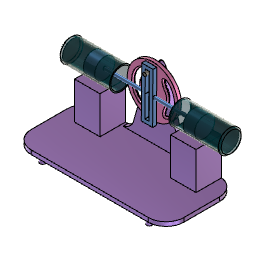
Yoke Mechanism (Autodesk Fusion 360 design; units mm, degrees)
Autodesk Fusion 360 part; units mm, degrees
note: some values were not read from the file. Set by a fixed rule: which face or edge a step refers to.
sketch "stand bottom" plane through (0, 0, 0) normal (0, 0, 1) x (1, 0, 0) in component "Stand"
  line L0 (150, 70) -> (-150, 70)
  line L1 (-150, 70) -> (-150, -70)
  line L2 (-150, -70) -> (150, -70)
  line L3 (150, -70) -> (150, 70)
  circle A0 centre (-105, 58) radius 5
  circle A1 centre (-105, -58) radius 5
  circle A2 centre (105, 58) radius 5
  circle A3 centre (105.0261, -58) radius 5
  dimension "d1" = 10
  dimension "d4" = 10
  dimension "d5" = 10
  dimension "d6" = 10
  constraint horizontal L0
  constraint vertical L1
  constraint horizontal L2
  constraint vertical L3
  measures "d1" diameter of A0
  measures "d4" diameter of A1
  measures "d5" diameter of A2
  measures "d6" diameter of A3
extrude "Extrude1" add sketch "stand bottom" along normal blind 8 contours L0 L1 L2 L3 | A0 | A1 | A2 | A3 makes body 1 in component "Stand"
extrude "Extrude2" add sketch "stand bottom" against normal blind 14 contours A0 | A1 | A2 | A3 bodies 1 in component "Stand"
fillet "Fillet1" radius 35 4 edges at (-150, 70, 4) (150, 70, 4) (150, -70, 4) (-150, -70, 4) on bodies 1 in component "Stand"
sketch "stand top" plane through (0, 70, 0) normal (0, 1, 0) x (-1, 0, 0) in component "Stand"
  line L0 (-115, 8) -> (-115, 0)
  line L1 (-115, 0) -> (115, 0)
  line L2 (115, 0) -> (115, 8)
  line L3 (115, 8) -> (-115, 8)
  line L4 (-50, 8) -> (50, 8)
  line L5 (-1.9252, 149.8221) -> (-2.2092, 149.8221)
  spline S0 degree 5 poles (-64.9527, 8) (-64.3612, 8.1995) (-63.1954, 8.61) (-61.498, 9.2603) (-59.339, 10.1978) (-56.826, 11.4952) (-54.5169, 12.9303) (-52.4304, 14.5157) (-50.5804, 16.2608) (-48.9632, 18.1632) (-47.5635, 20.2124) (-46.6045, 21.9603) (-45.9702, 23.3287) (-45.5844, 24.2659) (-45.4008, 24.7409) knots 0 0 0 0 0 0 0.1 0.2 0.3 0.4 0.5 0.6 0.7 0.8 0.9 1 1 1 1 1 1
  spline S1 degree 5 poles (65.0799, 8) (64.5003, 8.2031) (63.3571, 8.6206) (61.69, 9.2805) (59.5642, 10.2292) (57.0799, 11.5375) (54.785, 12.98) (52.6968, 14.5689) (50.8278, 16.3131) (49.1739, 18.2095) (47.7205, 20.248) (46.7061, 21.9839) (46.0235, 23.3412) (45.6026, 24.2703) (45.4008, 24.7409) knots 0 0 0 0 0 0 0.1 0.2 0.3 0.4 0.5 0.6 0.7 0.8 0.9 1 1 1 1 1 1
  line L6 (-64.9527, 8) -> (65.0799, 8)
  spline S2 degree 5 poles (-45.4008, 24.7409) (-42.8881, 33.5033) (-38.082, 50.4523) (-31.5308, 74.1483) (-24.0174, 102.0268) (-16.1362, 129.1634) (-9.099, 146.6861) (-2.2181, 152.8633) (5.106, 146.8269) (13.2741, 129.4242) (22.5509, 102.341) (30.9962, 74.4151) (37.9521, 50.6146) (42.871, 33.5629) (45.4008, 24.7408) knots 0 0 0 0 0 0 0.1 0.2 0.3 0.4 0.5 0.6 0.7 0.8 0.9 1 1 1 1 1 1
  line L7 (-51.345, 4.0119) -> (-39.4565, 45.4698)
  line L8 (39.4565, 45.4698) -> (51.345, 4.0119)
  point P0 (-51.9875, 14.9922)
  point P1 (52.3054, 14.9922)
  dimension "d14" = 100
  constraint horizontal L4
  constraint horizontal L5
  constraint coincident L3 S0.start
  constraint coincident L3 S1.start
  constraint coincident S1.end S2
  constraint coincident S1 S2.end
  constraint midpoint S0.end L7
  constraint midpoint S2.end L8
  constraint coincident S2 L5.start
  measures "d14" distance of L4.start L4.end
extrude "Extrude3" add sketch "stand top" against normal blind 10 contours L3 S0 L6 L7 | L3 L4 L5 L6 S2 L7 L8 | L3 S1 L6 L8 bodies 1 in component "Stand"
sketch "crank holes" plane through (0, 60, 0) normal (0, -1, 0) x (1, 0, 0) in component "Crank"
  line L0 (-65.0799, 8) -> (64.9527, 8)
  spline S0 degree 5 poles (64.9527, 8) (64.3612, 8.1995) (63.1954, 8.61) (61.498, 9.2603) (59.339, 10.1978) (56.826, 11.4952) (54.5169, 12.9303) (52.4304, 14.5157) (50.5804, 16.2608) (48.9632, 18.1632) (47.5635, 20.2124) (46.6045, 21.9603) (45.9702, 23.3287) (45.5844, 24.2659) (45.4008, 24.7409) knots 0 0 0 0 0 0 0.1 0.2 0.3 0.4 0.5 0.6 0.7 0.8 0.9 1 1 1 1 1 1
  spline S1 degree 5 poles (45.4008, 24.7409) (42.8881, 33.5033) (38.082, 50.4523) (31.5308, 74.1483) (24.0174, 102.0268) (16.1583, 129.0872) (10.546, 143.0831) (6.4127, 148.5135) (3.6169, 149.7753) (2.2092, 149.8221) knots 0 0 0 0 0 0 0.1 0.2 0.3 0.4 0.498596 0.498596 0.498596 0.498596 0.498596 0.498596
  line L1 (2.2092, 149.8221) -> (1.9252, 149.8221)
  spline S2 degree 5 poles (-45.4008, 24.7409) (-45.6026, 24.2703) (-46.0235, 23.3412) (-46.7061, 21.9839) (-47.7205, 20.248) (-49.1739, 18.2095) (-50.8278, 16.3131) (-52.6968, 14.5689) (-54.785, 12.98) (-57.0799, 11.5375) (-59.5642, 10.2292) (-61.69, 9.2805) (-63.3571, 8.6206) (-64.5003, 8.2031) (-65.0799, 8) knots -1 -1 -1 -1 -1 -1 -0.9 -0.8 -0.7 -0.6 -0.5 -0.4 -0.3 -0.2 -0.1 0 0 0 0 0 0
  spline S3 degree 5 poles (-30, 90) (-30.1222, 90.4299) (-30.1922, 91.398) (-29.7437, 93.1541) (-27.9759, 95.973) (-23.8911, 99.8217) (-18.1874, 103.4577) (-11.2539, 106.3526) (-3.5648, 108.0684) (4.367, 108.3276) (12.0396, 107.1126) (18.9937, 104.6588) (24.8283, 101.3641) (29.2216, 97.7238) (31.9508, 94.2565) (32.9127, 91.4333) (32.146, 89.6068) (29.8541, 88.9368) (26.3462, 89.3976) (21.972, 90.7776) (17.0724, 92.7047) (11.9619, 94.7305) (6.9054, 96.4005) (2.0938, 97.3326) (-2.3738, 97.2842) (-6.5262, 96.2467) (-10.4934, 94.4463) (-14.4197, 92.253) (-18.388, 90.114) (-22.3503, 88.4802) (-26.0299, 87.7313) (-28.3367, 88.0383) (-29.4588, 88.8188) (-29.8778, 89.5701) (-30, 90) knots 0 0 0 0 0 0 0.033333 0.066667 0.1 0.133333 0.166667 0.2 0.233333 0.266667 0.3 0.333333 0.366667 0.4 0.433333 0.466667 0.5 0.533333 0.566667 0.6 0.633333 0.666667 0.7 0.733333 0.766667 0.8 0.833333 0.866667 0.9 0.933333 0.966667 1 1 1 1 1 1
  spline S4 degree 5 poles (31.4369, 46.3788) (31.5413, 45.9359) (31.5774, 44.9363) (31.0882, 43.1175) (29.2976, 40.1923) (25.2372, 36.2169) (19.5947, 32.514) (12.737, 29.663) (5.1206, 28.1374) (-2.7442, 28.2233) (-10.33, 29.9039) (-17.1277, 32.8669) (-22.6835, 36.6203) (-26.6352, 40.5748) (-28.7502, 44.14) (-28.9632, 46.8127) (-27.4177, 48.2723) (-24.5009, 48.4663) (-20.7069, 47.5475) (-16.5203, 45.8198) (-12.2699, 43.683) (-8.1234, 41.5748) (-4.1345, 39.9118) (-0.2722, 39.028) (3.5427, 39.1206) (7.4052, 40.1744) (11.3918, 41.9656) (15.5288, 44.1399) (19.7568, 46.269) (23.902, 47.9142) (27.6282, 48.6884) (29.8854, 48.3891) (30.9509, 47.5938) (31.3325, 46.8217) (31.4369, 46.3788) knots 0 0 0 0 0 0 0.033333 0.066667 0.1 0.133333 0.166667 0.2 0.233333 0.266667 0.3 0.333333 0.366667 0.4 0.433333 0.466667 0.5 0.533333 0.566667 0.6 0.633333 0.666667 0.7 0.733333 0.766667 0.8 0.833333 0.866667 0.9 0.933333 0.966667 1 1 1 1 1 1
  spline S5 degree 5 poles (1.9252, 149.8221) (0.531, 149.7759) (-2.3348, 148.5351) (-6.8236, 143.1672) (-13.3217, 129.285) (-22.5509, 102.341) (-30.9962, 74.4151) (-37.9521, 50.6146) (-42.871, 33.5629) (-45.4008, 24.7409) knots 0.50257 0.50257 0.50257 0.50257 0.50257 0.50257 0.6 0.7 0.8 0.9 1 1 1 1 1 1
  point P0 (0, 108)
  point P1 (32.484, 91.6271)
  point P2 (27.3786, 89.3794)
  point P3 (-0.1137, 97.1853)
  point P4 (-21.072, 89.1079)
  point P5 (-28.5631, 46.3788)
  point P6 (-19.4459, 46.9397)
  point P7 (1.4369, 28.3788)
  point P8 (22.5089, 47.2709)
  point P9 (1.5506, 39.1935)
  constraint coincident S1 P2
sketch "crank" plane through (0, 60, 0) normal (0, -1, 0) x (1, 0, 0) in component "Crank"
  circle A0 centre (0.0497, 67.3306) radius 50
  dimension "d19" = 100
  measures "d19" diameter of A0
extrude "Extrude1'" add sketch "crank" along normal blind 6.5 separate body makes body 2 in component "Crank"
extrude "Extrude2'" cut sketch "crank holes" along normal blind 20 contours S1 S3 S5 | S3 S5 | S1 S3 | S4 bodies 2 in component "Crank"
fillet "Fillet1'" radius 2.5 1 faces at (19.1682, 57.8333, 91.8987) on bodies 2 in component "Crank"
fillet "Fillet2" radius 2.5 1 faces at (12.9137, 55.6667, 42.7911) on bodies 2 in component "Crank"
sketch "crank pin" plane through (0, 53.5, 0) normal (0, -1, 0) x (1, 0, 0) in component "Crank"
  spline S0 degree 3 poles (-32.4047, 89.3162) (-32.2002, 88.597) (-31.8287, 87.9253) (-30.5196, 86.4929) (-29.397, 85.9429) (-27.7418, 85.5869) (-27.2429, 85.5296) (-25.5741, 85.4613) (-24.4031, 85.6084) (-22.117, 86.1062) (-20.9991, 86.4599) (-18.0884, 87.5643) (-16.3403, 88.4246) (-12.8647, 90.2551) (-11.1373, 91.2339) (-8.0614, 92.7587) (-6.7334, 93.3488) (-3.982, 94.2439) (-2.5577, 94.5401) (0.5399, 94.7607) (2.2064, 94.6297) (6.2945, 93.9154) (8.6805, 93.1627) (12.6221, 91.7573) (14.2021, 91.1432) (17.2778, 89.946) (18.7736, 89.3612) (21.6215, 88.3307) (22.9694, 87.8752) (25.3002, 87.237) (26.2721, 87.0129) (28.5577, 86.6781) (29.8981, 86.6164) (31.6823, 87.0406) (32.1742, 87.2205) (33.458, 87.9311) (34.1502, 88.6448) (34.8897, 90.2302) (35.0207, 91.0446) (34.9052, 93.1494) (34.4037, 94.3994) (32.8586, 97.0913) (31.6734, 98.4685) (29.0957, 100.9728) (27.6888, 102.0975) (22.8051, 105.4634) (19.0241, 107.252) (11.0474, 109.7644) (6.8251, 110.452) (-0.3594, 110.5842) (-3.3171, 110.3429) (-9.1325, 109.2942) (-11.9883, 108.4886) (-16.7168, 106.6518) (-18.6397, 105.7493) (-21.906, 103.9112) (-23.2799, 103.0321) (-25.4581, 101.4258) (-26.2992, 100.7465) (-27.9744, 99.2379) (-28.8028, 98.401) (-30.1414, 96.809) (-30.6813, 96.079) (-31.4524, 94.8032) (-31.7251, 94.2831) (-32.2133, 93.1239) (-32.4148, 92.4775) (-32.6035, 91.3035) (-32.6287, 90.7829) (-32.5513, 89.9463) (-32.4931, 89.627) (-32.4047, 89.3162) knots -36.87303517 -36.87303517 -36.87303517 -36.87303517 -36.59704222 -36.59704222 -36.15680654 -36.15680654 -35.97209665 -35.97209665 -35.54026559 -35.54026559 -35.10843452 -35.10843452 -34.39112682 -34.39112682 -33.65770849 -33.65770849 -33.12392068 -33.12392068 -32.59012672 -32.59012672 -31.97764095 -31.97764095 -31.05827941 -31.05827941 -30.43187642 -30.43187642 -29.83920987 -29.83920987 -29.31415769 -29.31415769 -28.94687666 -28.94687666 -28.4615352 -28.4615352 -28.26997051 -28.26997051 -27.91990285 -27.91990285 -27.62431801 -27.62431801 -27.14178902 -27.14178902 -26.47846917 -26.47846917 -25.81514933 -25.81514933 -24.2891365 -24.2891365 -22.72668726 -22.72668726 -21.63678991 -21.63678991 -20.54546925 -20.54546925 -19.76392124 -19.76392124 -19.16273047 -19.16273047 -18.76364224 -18.76364224 -18.33039407 -18.33039407 -17.99617584 -17.99617584 -17.77997858 -17.77997858 -17.53188563 -17.53188563 -17.34104489 -17.34104489 -17.22176943 -17.22176943 -17.22176943 -17.22176943
  circle A0 centre (0.0497, 67.3306) radius 50
  spline S1 degree 3 poles (33.8702, 46.9525) (33.7673, 47.3887) (33.6068, 47.8118) (33.0061, 48.8977) (32.4431, 49.4885) (31.0994, 50.3592) (30.3223, 50.6347) (28.791, 50.9139) (28.0381, 50.9408) (26.3548, 50.8495) (25.4262, 50.694) (22.2649, 49.9512) (20.1088, 49.0782) (16.5392, 47.4347) (15.095, 46.7026) (12.1973, 45.2273) (10.7441, 44.4811) (8.5258, 43.4711) (7.7841, 43.1548) (5.7652, 42.3957) (4.4602, 42.0117) (2.2222, 41.6956) (1.31, 41.6594) (-0.503, 41.7823) (-1.402, 41.9396) (-4.2235, 42.6592) (-6.0723, 43.4581) (-9.5174, 45.0826) (-11.1252, 45.9081) (-13.7245, 47.1836) (-14.7078, 47.6541) (-17.001, 48.6799) (-18.3199, 49.2195) (-20.5724, 49.97) (-21.4888, 50.2307) (-23.3369, 50.6129) (-24.2699, 50.7381) (-26.2035, 50.747) (-27.2125, 50.6101) (-28.6325, 50.0197) (-29.1022, 49.7395) (-30.014, 48.9559) (-30.4226, 48.4155) (-30.9212, 47.3276) (-31.0582, 46.8033) (-31.1858, 45.5883) (-31.1253, 44.8947) (-30.7455, 43.198) (-30.3147, 42.225) (-29.4705, 40.7504) (-29.1117, 40.21) (-27.8354, 38.4776) (-26.8112, 37.369) (-23.6636, 34.4157) (-21.3575, 32.7687) (-15.5428, 29.4373) (-11.8892, 27.9817) (-5.984, 26.5351) (-3.8202, 26.1833) (1.6474, 25.744) (4.9692, 25.8858) (10.4357, 26.7953) (12.6173, 27.3464) (16.9342, 28.8183) (19.0646, 29.7497) (22.5636, 31.6522) (23.9796, 32.5395) (26.5538, 34.4097) (27.7243, 35.3757) (29.5534, 37.1373) (30.2557, 37.8879) (31.5452, 39.4688) (32.1351, 40.2986) (33.0522, 41.9092) (33.4076, 42.6746) (33.8719, 44.1661) (34.0067, 44.8845) (34.0192, 46.0595) (33.9739, 46.5126) (33.8702, 46.9525) knots -50.17481759 -50.17481759 -50.17481759 -50.17481759 -49.94582152 -49.94582152 -49.54091284 -49.54091284 -49.12785412 -49.12785412 -48.74565958 -48.74565958 -48.26666293 -48.26666293 -47.08607969 -47.08607969 -46.25822908 -46.25822908 -45.4243524 -45.4243524 -45.01222338 -45.01222338 -44.32140201 -44.32140201 -43.85749851 -43.85749851 -43.39359501 -43.39359501 -42.36995809 -42.36995809 -41.44707773 -41.44707773 -40.88986856 -40.88986856 -40.16336921 -40.16336921 -39.67695209 -39.67695209 -39.19871179 -39.19871179 -38.68910161 -38.68910161 -38.41314855 -38.41314855 -38.07490321 -38.07490321 -37.80173618 -37.80173618 -37.45077222 -37.45077222 -36.91346781 -36.91346781 -36.58272177 -36.58272177 -35.81423378 -35.81423378 -34.37765011 -34.37765011 -32.38849479 -32.38849479 -31.27192126 -31.27192126 -29.58592663 -29.58592663 -28.44053696 -28.44053696 -27.25640945 -27.25640945 -26.40408789 -26.40408789 -25.6313644 -25.6313644 -25.10672795 -25.10672795 -24.58857947 -24.58857947 -24.15996572 -24.15996572 -23.79053685 -23.79053685 -23.5596438 -23.5596438 -23.5596438 -23.5596438
  circle A1 centre (-36.403, 67.3306) radius 4
  arc A2 (31.9944, 49.771) -> (31.9946, 49.7712) centre (0.0497, 67.3306) ccw
  arc A3 (30.8161, 86.8814) -> (30.816, 86.8814) centre (0.0497, 67.3306) ccw
  dimension "d28" = 8
  constraint coincident S1 A2.end
  constraint coincident S0 A3.start
  constraint coincident S1 A2.start
  constraint coincident S0 A3.end
  measures "d28" diameter of A1
extrude "Extrude3'" add sketch "crank pin" along normal blind 16 and the other way blind 5 separate body contours A1 A2 A3 | A1 A2 A3 makes body 3 in component "Crank"
sketch "stand pin" plane through (0, 60, 0) normal (0, -1, 0) x (1, 0, 0) in component "Stand"
  line L0 (-65.0799, 8) -> (64.9527, 8)
  spline S0 degree 5 poles (64.9527, 8) (64.3612, 8.1995) (63.1954, 8.61) (61.498, 9.2603) (59.339, 10.1978) (56.826, 11.4952) (54.5169, 12.9303) (52.4304, 14.5157) (50.5804, 16.2608) (48.9632, 18.1632) (47.5635, 20.2124) (46.6045, 21.9603) (45.9702, 23.3287) (45.5844, 24.2659) (45.4008, 24.7409) knots 0 0 0 0 0 0 0.1 0.2 0.3 0.4 0.5 0.6 0.7 0.8 0.9 1 1 1 1 1 1
  spline S1 degree 5 poles (45.4008, 24.7409) (42.8881, 33.5033) (38.082, 50.4523) (31.5308, 74.1483) (24.0174, 102.0268) (16.1583, 129.0872) (10.546, 143.0831) (6.4127, 148.5135) (3.6169, 149.7753) (2.2092, 149.8221) knots 0 0 0 0 0 0 0.1 0.2 0.3 0.4 0.498596 0.498596 0.498596 0.498596 0.498596 0.498596
  line L1 (2.2092, 149.8221) -> (1.9252, 149.8221)
  spline S2 degree 5 poles (-45.4008, 24.7409) (-45.6026, 24.2703) (-46.0235, 23.3412) (-46.7061, 21.9839) (-47.7205, 20.248) (-49.1739, 18.2095) (-50.8278, 16.3131) (-52.6968, 14.5689) (-54.785, 12.98) (-57.0799, 11.5375) (-59.5642, 10.2292) (-61.69, 9.2805) (-63.3571, 8.6206) (-64.5003, 8.2031) (-65.0799, 8) knots -1 -1 -1 -1 -1 -1 -0.9 -0.8 -0.7 -0.6 -0.5 -0.4 -0.3 -0.2 -0.1 0 0 0 0 0 0
  circle A0 centre (1.5, 104) radius 3
  spline S3 degree 5 poles (1.9252, 149.8221) (0.531, 149.7759) (-2.3348, 148.5351) (-6.8236, 143.1672) (-13.3217, 129.285) (-22.5509, 102.341) (-30.9962, 74.4151) (-37.9521, 50.6146) (-42.871, 33.5629) (-45.4008, 24.7409) knots 0.50257 0.50257 0.50257 0.50257 0.50257 0.50257 0.6 0.7 0.8 0.9 1 1 1 1 1 1
  dimension "d34" = 6
  measures "d34" diameter of A0
extrude "Extrude4" cut sketch "stand pin" against normal blind 0.7 bodies 1 in component "Stand"
extrude "Extrude5" add 1 faces at (3.554, 60, 103.4545) along direction (0, -1, 0) blind 10 and the other way blind 10 on bodies 1 bodies 1 in component "Stand"
sketch "crank middle hole" plane through (0, 53.5, 0) normal (0, -1, 0) x (1, 0, 0) in component "Crank"
  spline S0 degree 3 poles (-32.4047, 89.3162) (-32.2002, 88.597) (-31.8287, 87.9253) (-30.5196, 86.4929) (-29.397, 85.9429) (-27.7418, 85.5869) (-27.2429, 85.5296) (-25.5741, 85.4613) (-24.4031, 85.6084) (-22.117, 86.1062) (-20.9991, 86.4599) (-18.0884, 87.5643) (-16.3403, 88.4246) (-12.8647, 90.2551) (-11.1373, 91.2339) (-8.0614, 92.7587) (-6.7334, 93.3488) (-3.982, 94.2439) (-2.5577, 94.5401) (0.5399, 94.7607) (2.2064, 94.6297) (6.2945, 93.9154) (8.6805, 93.1627) (12.6221, 91.7573) (14.2021, 91.1432) (17.2778, 89.946) (18.7736, 89.3612) (21.6215, 88.3307) (22.9694, 87.8752) (25.3002, 87.237) (26.2721, 87.0129) (28.5577, 86.6781) (29.8981, 86.6164) (31.6823, 87.0406) (32.1742, 87.2205) (33.458, 87.9311) (34.1502, 88.6448) (34.8897, 90.2302) (35.0207, 91.0446) (34.9052, 93.1494) (34.4037, 94.3994) (32.8586, 97.0913) (31.6734, 98.4685) (29.0957, 100.9728) (27.6888, 102.0975) (22.8051, 105.4634) (19.0241, 107.252) (11.0474, 109.7644) (6.8251, 110.452) (-0.3594, 110.5842) (-3.3171, 110.3429) (-9.1325, 109.2942) (-11.9883, 108.4886) (-16.7168, 106.6518) (-18.6397, 105.7493) (-21.906, 103.9112) (-23.2799, 103.0321) (-25.4581, 101.4258) (-26.2992, 100.7465) (-27.9744, 99.2379) (-28.8028, 98.401) (-30.1414, 96.809) (-30.6813, 96.079) (-31.4524, 94.8032) (-31.7251, 94.2831) (-32.2133, 93.1239) (-32.4148, 92.4775) (-32.6035, 91.3035) (-32.6287, 90.7829) (-32.5513, 89.9463) (-32.4931, 89.627) (-32.4047, 89.3162) knots -36.87303517 -36.87303517 -36.87303517 -36.87303517 -36.59704222 -36.59704222 -36.15680654 -36.15680654 -35.97209665 -35.97209665 -35.54026559 -35.54026559 -35.10843452 -35.10843452 -34.39112682 -34.39112682 -33.65770849 -33.65770849 -33.12392068 -33.12392068 -32.59012672 -32.59012672 -31.97764095 -31.97764095 -31.05827941 -31.05827941 -30.43187642 -30.43187642 -29.83920987 -29.83920987 -29.31415769 -29.31415769 -28.94687666 -28.94687666 -28.4615352 -28.4615352 -28.26997051 -28.26997051 -27.91990285 -27.91990285 -27.62431801 -27.62431801 -27.14178902 -27.14178902 -26.47846917 -26.47846917 -25.81514933 -25.81514933 -24.2891365 -24.2891365 -22.72668726 -22.72668726 -21.63678991 -21.63678991 -20.54546925 -20.54546925 -19.76392124 -19.76392124 -19.16273047 -19.16273047 -18.76364224 -18.76364224 -18.33039407 -18.33039407 -17.99617584 -17.99617584 -17.77997858 -17.77997858 -17.53188563 -17.53188563 -17.34104489 -17.34104489 -17.22176943 -17.22176943 -17.22176943 -17.22176943
  circle A0 centre (0.0497, 67.3306) radius 50
  spline S1 degree 3 poles (33.8702, 46.9525) (33.7673, 47.3887) (33.6068, 47.8118) (33.0061, 48.8977) (32.4431, 49.4885) (31.0994, 50.3592) (30.3223, 50.6347) (28.791, 50.9139) (28.0381, 50.9408) (26.3548, 50.8495) (25.4262, 50.694) (22.2649, 49.9512) (20.1088, 49.0782) (16.5392, 47.4347) (15.095, 46.7026) (12.1973, 45.2273) (10.7441, 44.4811) (8.5258, 43.4711) (7.7841, 43.1548) (5.7652, 42.3957) (4.4602, 42.0117) (2.2222, 41.6956) (1.31, 41.6594) (-0.503, 41.7823) (-1.402, 41.9396) (-4.2235, 42.6592) (-6.0723, 43.4581) (-9.5174, 45.0826) (-11.1252, 45.9081) (-13.7245, 47.1836) (-14.7078, 47.6541) (-17.001, 48.6799) (-18.3199, 49.2195) (-20.5724, 49.97) (-21.4888, 50.2307) (-23.3369, 50.6129) (-24.2699, 50.7381) (-26.2035, 50.747) (-27.2125, 50.6101) (-28.6325, 50.0197) (-29.1022, 49.7395) (-30.014, 48.9559) (-30.4226, 48.4155) (-30.9212, 47.3276) (-31.0582, 46.8033) (-31.1858, 45.5883) (-31.1253, 44.8947) (-30.7455, 43.198) (-30.3147, 42.225) (-29.4705, 40.7504) (-29.1117, 40.21) (-27.8354, 38.4776) (-26.8112, 37.369) (-23.6636, 34.4157) (-21.3575, 32.7687) (-15.5428, 29.4373) (-11.8892, 27.9817) (-5.984, 26.5351) (-3.8202, 26.1833) (1.6474, 25.744) (4.9692, 25.8858) (10.4357, 26.7953) (12.6173, 27.3464) (16.9342, 28.8183) (19.0646, 29.7497) (22.5636, 31.6522) (23.9796, 32.5395) (26.5538, 34.4097) (27.7243, 35.3757) (29.5534, 37.1373) (30.2557, 37.8879) (31.5452, 39.4688) (32.1351, 40.2986) (33.0522, 41.9092) (33.4076, 42.6746) (33.8719, 44.1661) (34.0067, 44.8845) (34.0192, 46.0595) (33.9739, 46.5126) (33.8702, 46.9525) knots -50.17481759 -50.17481759 -50.17481759 -50.17481759 -49.94582152 -49.94582152 -49.54091284 -49.54091284 -49.12785412 -49.12785412 -48.74565958 -48.74565958 -48.26666293 -48.26666293 -47.08607969 -47.08607969 -46.25822908 -46.25822908 -45.4243524 -45.4243524 -45.01222338 -45.01222338 -44.32140201 -44.32140201 -43.85749851 -43.85749851 -43.39359501 -43.39359501 -42.36995809 -42.36995809 -41.44707773 -41.44707773 -40.88986856 -40.88986856 -40.16336921 -40.16336921 -39.67695209 -39.67695209 -39.19871179 -39.19871179 -38.68910161 -38.68910161 -38.41314855 -38.41314855 -38.07490321 -38.07490321 -37.80173618 -37.80173618 -37.45077222 -37.45077222 -36.91346781 -36.91346781 -36.58272177 -36.58272177 -35.81423378 -35.81423378 -34.37765011 -34.37765011 -32.38849479 -32.38849479 -31.27192126 -31.27192126 -29.58592663 -29.58592663 -28.44053696 -28.44053696 -27.25640945 -27.25640945 -26.40408789 -26.40408789 -25.6313644 -25.6313644 -25.10672795 -25.10672795 -24.58857947 -24.58857947 -24.15996572 -24.15996572 -23.79053685 -23.79053685 -23.5596438 -23.5596438 -23.5596438 -23.5596438
  circle A1 centre (0.0497, 67.3306) radius 3
  dimension "d41" = 6
  constraint concentric A0 A1
  measures "d41" diameter of A1
extrude "Extrude4'" cut 1 faces at (3.554, 50, 103.4545) along direction (0, 1, 0) blind 100 on bodies 1 bodies 3 2 in component "Crank"
move_face "OffsetFaces1" offset -0.3 1 faces at (4.3191, 57.1333, 102.9739) on bodies 1 in component "Stand"
sketch "left cylinder" plane through (-150, 0, 0) normal (-1, 0, 0) x (0, -1, 0) in component "Cylinders"
  line L0 (35, 0) -> (35, 8)
  line L1 (35, 8) -> (-35, 8)
  line L2 (-35, 8) -> (-35, 0)
  line L3 (-35, 0) -> (35, 0)
  circle A0 centre (10, 70) radius 22.5
  dimension "d45" = 45
  measures "d45" diameter of A0
extrude "Extrude1''" add sketch "left cylinder" against normal blind 100 separate body contours A0 makes body 4 in component "Cylinders"
sketch "left cylinder hole" plane through (-50, 0, 0) normal (1, 0, 0) x (0, 1, 0) in component "Cylinders"
  circle A0 centre (-10, 70) radius 22.5
  circle A1 centre (-10, 70) radius 20
  dimension "d48" = 40
  constraint concentric A0 A1
  measures "d48" diameter of A1
extrude "Extrude2''" cut sketch "left cylinder hole" against normal blind 95 contours A1 bodies 4 in component "Cylinders"
sketch "right cylinder" plane through (130.7682, 0, 0) normal (1, 0, 0) x (0, 1, 0) in component "Cylinders"
  line L0 (-66.6038, 25.1959) -> (-66.6038, 17.1959)
  line L1 (-66.6038, 17.1959) -> (3.3962, 17.1959)
  line L2 (3.3962, 17.1959) -> (3.3962, 25.1959)
  line L3 (3.3962, 25.1959) -> (-66.6038, 25.1959)
  circle A0 centre (-10, 70) radius 22.5
  dimension "d51" = 45
  measures "d51" diameter of A0
extrude "Extrude3''" add sketch "right cylinder" against normal blind 100 separate body contours A0 makes body 5 in component "Cylinders"
sketch "right cylinder hole" plane through (30.7682, 0, 0) normal (-1, 0, 0) x (0, -1, 0) in component "Cylinders"
  circle A0 centre (10, 70) radius 22.5
  circle A1 centre (10, 70) radius 20
  dimension "d54" = 40
  constraint concentric A0 A1
  measures "d54" diameter of A1
extrude "Extrude4''" cut sketch "right cylinder hole" against normal blind 95 contours A1 bodies 5 in component "Cylinders"
sketch "piston middle" plane through (0, 53.5, 0) normal (0, -1, 0) x (1, 0, 0) in component "Piston"
  spline S0 degree 3 poles (-32.4047, 89.3162) (-32.2002, 88.597) (-31.8287, 87.9253) (-30.5196, 86.4929) (-29.397, 85.9429) (-27.7418, 85.5869) (-27.2429, 85.5296) (-25.5741, 85.4613) (-24.4031, 85.6084) (-22.117, 86.1062) (-20.9991, 86.4599) (-18.0884, 87.5643) (-16.3403, 88.4246) (-12.8647, 90.2551) (-11.1373, 91.2339) (-8.0614, 92.7587) (-6.7334, 93.3488) (-3.982, 94.2439) (-2.5577, 94.5401) (0.5399, 94.7607) (2.2064, 94.6297) (6.2945, 93.9154) (8.6805, 93.1627) (12.6221, 91.7573) (14.2021, 91.1432) (17.2778, 89.946) (18.7736, 89.3612) (21.6215, 88.3307) (22.9694, 87.8752) (25.3002, 87.237) (26.2721, 87.0129) (28.5577, 86.6781) (29.8981, 86.6164) (31.6823, 87.0406) (32.1742, 87.2205) (33.458, 87.9311) (34.1502, 88.6448) (34.8897, 90.2302) (35.0207, 91.0446) (34.9052, 93.1494) (34.4037, 94.3994) (32.8586, 97.0913) (31.6734, 98.4685) (29.0957, 100.9728) (27.6888, 102.0975) (22.8051, 105.4634) (19.0241, 107.252) (11.0474, 109.7644) (6.8251, 110.452) (-0.3594, 110.5842) (-3.3171, 110.3429) (-9.1325, 109.2942) (-11.9883, 108.4886) (-16.7168, 106.6518) (-18.6397, 105.7493) (-21.906, 103.9112) (-23.2799, 103.0321) (-25.4581, 101.4258) (-26.2992, 100.7465) (-27.9744, 99.2379) (-28.8028, 98.401) (-30.1414, 96.809) (-30.6813, 96.079) (-31.4524, 94.8032) (-31.7251, 94.2831) (-32.2133, 93.1239) (-32.4148, 92.4775) (-32.6035, 91.3035) (-32.6287, 90.7829) (-32.5513, 89.9463) (-32.4931, 89.627) (-32.4047, 89.3162) knots -36.87303517 -36.87303517 -36.87303517 -36.87303517 -36.59704222 -36.59704222 -36.15680654 -36.15680654 -35.97209665 -35.97209665 -35.54026559 -35.54026559 -35.10843452 -35.10843452 -34.39112682 -34.39112682 -33.65770849 -33.65770849 -33.12392068 -33.12392068 -32.59012672 -32.59012672 -31.97764095 -31.97764095 -31.05827941 -31.05827941 -30.43187642 -30.43187642 -29.83920987 -29.83920987 -29.31415769 -29.31415769 -28.94687666 -28.94687666 -28.4615352 -28.4615352 -28.26997051 -28.26997051 -27.91990285 -27.91990285 -27.62431801 -27.62431801 -27.14178902 -27.14178902 -26.47846917 -26.47846917 -25.81514933 -25.81514933 -24.2891365 -24.2891365 -22.72668726 -22.72668726 -21.63678991 -21.63678991 -20.54546925 -20.54546925 -19.76392124 -19.76392124 -19.16273047 -19.16273047 -18.76364224 -18.76364224 -18.33039407 -18.33039407 -17.99617584 -17.99617584 -17.77997858 -17.77997858 -17.53188563 -17.53188563 -17.34104489 -17.34104489 -17.22176943 -17.22176943 -17.22176943 -17.22176943
  circle A0 centre (0.0497, 67.3306) radius 50
  spline S1 degree 3 poles (33.8702, 46.9525) (33.7673, 47.3887) (33.6068, 47.8118) (33.0061, 48.8977) (32.4431, 49.4885) (31.0994, 50.3592) (30.3223, 50.6347) (28.791, 50.9139) (28.0381, 50.9408) (26.3548, 50.8495) (25.4262, 50.694) (22.2649, 49.9512) (20.1088, 49.0782) (16.5392, 47.4347) (15.095, 46.7026) (12.1973, 45.2273) (10.7441, 44.4811) (8.5258, 43.4711) (7.7841, 43.1548) (5.7652, 42.3957) (4.4602, 42.0117) (2.2222, 41.6956) (1.31, 41.6594) (-0.503, 41.7823) (-1.402, 41.9396) (-4.2235, 42.6592) (-6.0723, 43.4581) (-9.5174, 45.0826) (-11.1252, 45.9081) (-13.7245, 47.1836) (-14.7078, 47.6541) (-17.001, 48.6799) (-18.3199, 49.2195) (-20.5724, 49.97) (-21.4888, 50.2307) (-23.3369, 50.6129) (-24.2699, 50.7381) (-26.2035, 50.747) (-27.2125, 50.6101) (-28.6325, 50.0197) (-29.1022, 49.7395) (-30.014, 48.9559) (-30.4226, 48.4155) (-30.9212, 47.3276) (-31.0582, 46.8033) (-31.1858, 45.5883) (-31.1253, 44.8947) (-30.7455, 43.198) (-30.3147, 42.225) (-29.4705, 40.7504) (-29.1117, 40.21) (-27.8354, 38.4776) (-26.8112, 37.369) (-23.6636, 34.4157) (-21.3575, 32.7687) (-15.5428, 29.4373) (-11.8892, 27.9817) (-5.984, 26.5351) (-3.8202, 26.1833) (1.6474, 25.744) (4.9692, 25.8858) (10.4357, 26.7953) (12.6173, 27.3464) (16.9342, 28.8183) (19.0646, 29.7497) (22.5636, 31.6522) (23.9796, 32.5395) (26.5538, 34.4097) (27.7243, 35.3757) (29.5534, 37.1373) (30.2557, 37.8879) (31.5452, 39.4688) (32.1351, 40.2986) (33.0522, 41.9092) (33.4076, 42.6746) (33.8719, 44.1661) (34.0067, 44.8845) (34.0192, 46.0595) (33.9739, 46.5126) (33.8702, 46.9525) knots -50.17481759 -50.17481759 -50.17481759 -50.17481759 -49.94582152 -49.94582152 -49.54091284 -49.54091284 -49.12785412 -49.12785412 -48.74565958 -48.74565958 -48.26666293 -48.26666293 -47.08607969 -47.08607969 -46.25822908 -46.25822908 -45.4243524 -45.4243524 -45.01222338 -45.01222338 -44.32140201 -44.32140201 -43.85749851 -43.85749851 -43.39359501 -43.39359501 -42.36995809 -42.36995809 -41.44707773 -41.44707773 -40.88986856 -40.88986856 -40.16336921 -40.16336921 -39.67695209 -39.67695209 -39.19871179 -39.19871179 -38.68910161 -38.68910161 -38.41314855 -38.41314855 -38.07490321 -38.07490321 -37.80173618 -37.80173618 -37.45077222 -37.45077222 -36.91346781 -36.91346781 -36.58272177 -36.58272177 -35.81423378 -35.81423378 -34.37765011 -34.37765011 -32.38849479 -32.38849479 -31.27192126 -31.27192126 -29.58592663 -29.58592663 -28.44053696 -28.44053696 -27.25640945 -27.25640945 -26.40408789 -26.40408789 -25.6313644 -25.6313644 -25.10672795 -25.10672795 -24.58857947 -24.58857947 -24.15996572 -24.15996572 -23.79053685 -23.79053685 -23.5596438 -23.5596438 -23.5596438 -23.5596438
  line L0 (-32.403, 80) -> (-32.403, 50)
  line L1 (-40.403, 80) -> (-40.403, 50)
  line L2 (-0.0105, 67.2019) -> (-36.403, 67.3306)
  circle A1 centre (-0.0105, 67.2019) radius 36.3928
  line L3 (-75, 103.5947) -> (90, 103.5947)
  line L4 (-70, 30.8091) -> (80, 30.8091)
  line L5 (-36.403, 67.3306) -> (-40.403, 67.3306)
  circle A2 centre (-0.0105, 67.2019) radius 40.3928
  line L6 (-70, 26.8091) -> (80, 26.8091)
  line L7 (-74.1733, 107.5946) -> (70, 107.5946)
  line L8 (-40.403, 24.523) -> (-32.2692, 24.523)
  line L9 (-32.2692, 24.523) -> (-32.2692, 109.881)
  line L10 (-32.2692, 109.881) -> (-40.403, 109.881)
  line L11 (-40.403, 109.881) -> (-40.403, 24.523)
  line L12 (-47.403, 17.523) -> (-25.2692, 17.523)
  line L13 (-25.2692, 17.523) -> (-25.2692, 116.881)
  line L14 (-25.2692, 116.881) -> (-47.403, 116.881)
  line L15 (-47.403, 116.881) -> (-47.403, 17.523)
  dimension "d57" = 4
  dimension "d58" = 85.358
  dimension "d59" = 7
  constraint vertical L0
  constraint vertical L1
  constraint coincident L2.start A1.centre
  constraint coincident L2.end A1
  constraint horizontal L3
  constraint horizontal L4
  constraint tangent A1 L4
  constraint tangent A1 L3
  constraint perpendicular L1 L5
  constraint concentric A1 A2
  constraint coincident L5.end A2
  constraint horizontal L6
  constraint parallel L3 L7
  constraint tangent A2 L7
  constraint tangent A2 L6
  constraint horizontal L8
  constraint vertical L9
  constraint horizontal L10
  constraint vertical L11
  measures "d57" distance of L2.end L5.end
  measures "d58" distance of L8.start L10.end
extrude "Extrude1'''" add sketch "piston middle" along normal blind 12.5 separate body contours S0 A1 A2 L9 L13 | S0 A1 L9 | S0 A1 L13 | S0 L2 A1 L9 L13 | S0 A2 L9 L13 | S0 L3 L9 L13 | A0 L1 L11 L15 | S1 L2 A1 L9 L13 | A0 L3 L7 L9 L13 | S1 A1 A2 L9 L13 | L4 A2 L9 L13 | A0 L7 L9 | A0 L3 L11 L15 | A0 L4 L11 L15 | A0 L4 L6 L9 L13 | S1 A1 L13 | S1 A1 L13 | A0 L7 L13 | L3 L7 L11 L15 | A0 L7 L9 L10 L11 L13 L14 L15 | L4 L6 L11 L15 | A0 L6 L9 | A0 L6 L8 L9 L11 L12 L13 L15 | A0 L6 L13 picked at (-27.4965, 88.658) picked at (-27.2127, 46.3884) picked at (-27.1588, 41.3571) makes body 6 in component "Piston"
move_face "OffsetFaces1'" offset -5 1 faces at (-45.0697, 53.5, 67.3306) on bodies 6 in component "Piston"
move_face "OffsetFaces1''" offset -0.3 1 faces at (-32.4229, 44.5, 67.7288) on bodies 3 in component "Crank"
sketch "piston left" plane through (-47.403, 0, 0) normal (-1, 0, 0) x (0, -1, 0) in component "Piston"
  line L0 (-48.5, 116.881) -> (-48.5, 17.523)
  line L1 (-48.5, 17.523) -> (-41, 17.523)
  line L2 (-41, 17.523) -> (-41, 116.881)
  line L3 (-41, 116.881) -> (-48.5, 116.881)
  circle A0 centre (-44.6997, 67.2631) radius 3.25
  dimension "d64" = 6.5
  measures "d64" diameter of A0
extrude "Extrude2'''" add sketch "piston left" along normal blind 75 contours A0 bodies 6 in component "Piston"
sketch "piston right" plane through (-25.2692, 0, 0) normal (1, 0, 0) x (0, 1, 0) in component "Piston"
  line L0 (48.5, 17.523) -> (48.5, 116.881)
  line L1 (48.5, 116.881) -> (41, 116.881)
  line L2 (41, 116.881) -> (41, 17.523)
  line L3 (41, 17.523) -> (48.5, 17.523)
  circle A0 centre (44.7028, 67.2408) radius 3.25
  dimension "d67" = 6.5
  measures "d67" diameter of A0
extrude "Extrude3'''" add sketch "piston right" along normal blind 75 contours A0 bodies 6 in component "Piston"
move_body "Move1" bodies 5 to x (1, 0, 0) y (0, 1, 0) z (0, 0, 1) at (-40, 0, 0) in component "Cylinders"
move_body "Move2" bodies 5 to x (1, 0, 0) y (0, 1, 0) z (0, 0, 1) at (14, 0, 0) in component "Cylinders"
move_body "Move3" bodies 5 to x (1, 0, 0) y (0, 1, 0) z (0, 0, 1) at (32, 0, 0) in component "Cylinders"
sketch "piston cover left" plane through (-122.403, 0, 0) normal (-1, 0, 0) x (0, -1, 0) in component "Piston"
  circle A0 centre (-44.6997, 67.2631) radius 3.25
  circle A1 centre (-44.6997, 67.2631) radius 19.75
  dimension "d70" = 39.5
  constraint concentric A0 A1
  measures "d70" diameter of A1
extrude "Extrude4'''" add sketch "piston cover left" along normal blind 23.3333 bodies 6 in component "Piston"
extrude "Extrude5'" add 1 faces at (-122.403, 45.4032, 66.3249) along direction (-1, 0, 0) blind 23.3333 on bodies 6 bodies 6 in component "Piston"
sketch "piston cover right" plane through (49.7308, 0, 0) normal (1, 0, 0) x (0, 1, 0) in component "Piston"
  circle A0 centre (44.7028, 67.2408) radius 3.25
  circle A1 centre (44.7028, 67.2408) radius 19.75
  dimension "d75" = 39.5
  constraint concentric A0 A1
  measures "d75" diameter of A1
extrude "Extrude6" add sketch "piston cover right" along normal blind 23.3333 contours A0 | A1 bodies 6 in component "Piston"
move_body "Move4" bodies 5 to x (1, 0, 0) y (0, 1, 0) z (0, 0, 1) at (30, 0, 0) in component "Cylinders"
fillet "Fillet1''" radius 3 1 edges at (-150, 10.9774, 61.8637) on bodies 4 in component "Cylinders"
fillet "Fillet2'" radius 3 1 edges at (166.7682, -30.9774, 61.8637) on bodies 5 in component "Cylinders"
move_face "OffsetFaces2" offset -1 1 faces at (49.7308, 58.8671, 66.0982) on bodies 6 in component "Piston"
move_face "OffsetFaces3" offset -1 1 faces at (-122.403, 30.5232, 68.2443) on bodies 6 in component "Piston"
move_face "OffsetFaces2'" offset -0.3 1 faces at (-32.7214, 44.5, 67.699) on bodies 3 in component "Crank"
sketch "stand holder for cylinders" plane through (0, 0, 8) normal (0, 0, 1) x (-1, 0, 0) in component "Stand"
  line L0 (65.0799, -60.7) -> (65.0799, -70)
  line L1 (65.0799, -70) -> (115, -70)
  arc A0 (115, -70) -> (150, -35) centre (115, -35) ccw
  line L2 (150, -35) -> (150, 35)
  arc A1 (150, 35) -> (115, 70) centre (115, 35) ccw
  line L3 (115, 70) -> (-115, 70)
  arc A2 (-115, 70) -> (-150, 35) centre (-115, 35) ccw
  line L4 (-150, 35) -> (-150, -35)
  arc A3 (-150, -35) -> (-115, -70) centre (-115, -35) ccw
  line L5 (-115, -70) -> (-64.9527, -70)
  line L6 (-64.9527, -70) -> (-64.9527, -60.7)
  line L7 (-64.9527, -60.7) -> (65.0799, -60.7)
  line L8 (70, -70) -> (120, -70)
  line L9 (120, -70) -> (120, -20)
  line L10 (120, -20) -> (70, -20)
  line L11 (70, -20) -> (70, -70)
  line L12 (-119.4517, -19.4678) -> (-119.4517, -69.4678)
  line L13 (-69.4517, -19.4678) -> (-119.4517, -19.4678)
  line L14 (-69.4517, -69.4678) -> (-69.4517, -19.4678)
  line L15 (-119.4517, -69.4678) -> (-69.4517, -69.4678)
  constraint horizontal L8
  constraint vertical L9
  constraint horizontal L10
  constraint vertical L11
  constraint coincident L1 L8.start
  constraint horizontal L15
  constraint vertical L14
  constraint horizontal L13
  constraint vertical L12
extrude "Extrude6'" add sketch "stand holder for cylinders" along normal blind 73.2428 contours L1 A0 L8 L9 L10 L11 | L12 L13 L14 L15 bodies 1 in component "Stand"
component "Stand" placed x (1, 0, 0) y (0, 1, 0) z (0, 0, 1) at (0.0004, -0.0439, -0.3501)
component "Crank" placed x (0, 0, -1) y (0, 1, 0) z (1, 0, 0) at (-66.1987, -1.0594, 104.7142)
component "Cylinders" placed x (1, 0, 0) y (0, 1, 0) z (0, 0, 1) at (-3.2934, 54.5872, 33.3924)
component "Piston" placed x (0.999974, 0, -0.00724) y (0, 1, 0) z (0.00724, 0, 0.999974) at (37.3761, 0.1906, 36.1762)
equation "d58 = 83.072 mm + 2.286 mm"
named bodies: "stand", "crank", "left cylinder", "right cylinder", "piston", "crank pin"
